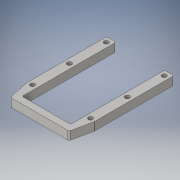
# Autodesk Inventor part: SpaceMX64
Saved by Autodesk Inventor 2016 (Build 200138000, 138)
## iProperties
Created: 2017-02-02
Part Number: SpaceMX64
Material: Generic
Document SubType Name: Modeling
Designer: Ghana
Density: 1 g/cm^3
Appearance: Default
Author: Ghana
Autodesk Inventor part; units mm, degrees
ref_plane "YZ Plane" through (0, 0, 0) normal (1, 0, 0) x (0, 1, 0)
ref_plane "XZ Plane" through (0, 0, 0) normal (0, 1, 0) x (-1, 0, 0)
ref_plane "XY Plane" through (0, 0, 0) normal (0, 0, 1) x (1, 0, 0)
sketch "Sketch2" plane through (0, 0, 0) normal (0, 1, 0) x (-1, 0, 0)
  line L0 (0.1834, -60.2221) -> (0.1834, -13.7487)
  line L1 (40.3834, -13.7487) -> (40.3834, -60.2221)
  line L2 (34.7834, -6.1497) -> (34.7834, -60.2221)
  line L3 (5.7834, -60.2221) -> (5.7834, -6.1497)
  circle A0 centre (37.5834, -14.2221) radius 1.35
  circle A1 centre (37.5834, -36.2221) radius 1.35
  circle A2 centre (2.9834, -14.2221) radius 1.35
  circle A3 centre (2.9834, -36.2221) radius 1.35
  circle A4 centre (37.5834, -58.2221) radius 1.35
  circle A5 centre (2.9834, -58.2221) radius 1.35
  line L4 (39.3834, -61.2221) -> (35.7834, -61.2221)
  line L5 (4.7834, -61.2221) -> (1.1834, -61.2221)
  line L6 (33.7834, -5.1497) -> (6.7834, -5.1497)
  arc A6 (34.7834, -6.1497) -> (33.7834, -5.1497) centre (33.7834, -6.1497) ccw
  arc A7 (6.7834, -5.1497) -> (5.7834, -6.1497) centre (6.7834, -6.1497) ccw
  arc A8 (39.3834, -61.2221) -> (40.3834, -60.2221) centre (39.3834, -60.2221) ccw
  arc A9 (34.7834, -60.2221) -> (35.7834, -61.2221) centre (35.7834, -60.2221) ccw
  arc A10 (4.7834, -61.2221) -> (5.7834, -60.2221) centre (4.7834, -60.2221) ccw
  arc A11 (0.1834, -60.2221) -> (1.1834, -61.2221) centre (1.1834, -60.2221) ccw
  line L7 (36.9709, -1.1834) -> (3.5958, -1.1834)
  line L8 (40.3623, -13.5445) -> (37.9499, -1.9792)
  line L9 (2.6169, -1.9792) -> (0.2044, -13.5445)
  arc A12 (40.3834, -13.7487) -> (40.3623, -13.5445) centre (39.3834, -13.7487) ccw
  arc A13 (37.9499, -1.9792) -> (36.9709, -1.1834) centre (36.9709, -2.1834) ccw
  arc A14 (3.5958, -1.1834) -> (2.6169, -1.9792) centre (3.5958, -2.1834) ccw
  arc A15 (0.2044, -13.5445) -> (0.1834, -13.7487) centre (1.1834, -13.7487) ccw
  constraints: 20 end point, 20 point on circle, 20 tangent, 16 centre point, 8 equal radius, 4 horizontal
extrude "Extrusion2" add sketch "Sketch2" along normal blind 5
body "Solid2"
